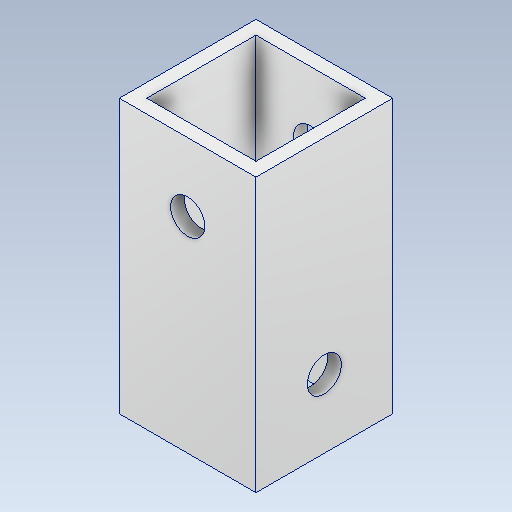
# Autodesk Inventor part: 前後直動12x12x24
Saved by Autodesk Inventor 2020.3 (Build 243373000, 373)
## iProperties
Created: 2020-07-05
Part Number: 前後直動12x12x24
Material: アルミニウム 6061
Document SubType Name: Modeling
Designer: totot
Density: 2.7 g/cm^3
Appearance: アルミニウム - フラット
Author: totot
Autodesk Inventor part; units mm, degrees
ref_plane "YZ Plane" through (0, 0, 0) normal (1, 0, 0) x (0, 1, 0)
ref_plane "XZ Plane" through (0, 0, 0) normal (0, 1, 0) x (-1, 0, 0)
ref_plane "XY Plane" through (0, 0, 0) normal (0, 0, 1) x (1, 0, 0)
sketch "スケッチ1" plane through (0, 0, 0) normal (0, 1, 0) x (-1, 0, 0)
  line L0 (0, 0) -> (12, 0)
  line L1 (12, 0) -> (12, -12)
  line L2 (12, -12) -> (0, -12)
  line L3 (0, -12) -> (0, 0)
  line L4 (1.2, -1.2) -> (10.8, -1.2)
  line L5 (10.8, -1.2) -> (10.8, -10.8)
  line L6 (10.8, -10.8) -> (1.2, -10.8)
  line L7 (1.2, -10.8) -> (1.2, -1.2)
  dimension "d0" = 12
  dimension "d1" = 12
  dimension "d2" = 9.6
  dimension "d3" = 9.6
  dimension "d4" = 1.2
  dimension "d5" = 1.2
  constraints: 16 end point, 4 parallel, 2 horizontal, 2 perpendicular
  measures "d0" distance of L1.end L2.end
  measures "d1" distance of L0.end L1.end
  measures "d2" distance of L5.end L6.end
  measures "d3" distance of L4.end L5.end
  measures "d4" distance between parallel lines of L0 L4
  measures "d5" distance between parallel lines of L7 L3
extrude "押し出し1" add sketch "スケッチ1" along normal blind 24
sketch "スケッチ2" plane through (-12, 0, -12) normal (-1, 0, 0) x (0, 0, 1)
  line L0 (0, 0) -> (12, 0) projected
  line L1 (0, 0) -> (0, 24) projected
  point P0 (6, 6)
  dimension "d8" = 6
  dimension "d9" = 6
  measures "d8" distance from line of point (6, 6) L0
  measures "d9" distance from line of L1 point (6, 6)
hole "穴1" at (-12, 6, -6) direction (1, 0, 0) diameter 3 end through all
sketch "スケッチ3" plane through (0, 0, -12) normal (0, 0, -1) x (-1, 0, 0)
  line L0 (0, 0) -> (0, 24) projected
  line L1 (0, 24) -> (12, 24) projected
  point P0 (6, 18)
  dimension "d17" = 6
  dimension "d18" = 6
  measures "d17" distance from line of L0 point (6, 18)
  measures "d18" distance from line of L1 point (6, 18)
hole "穴2" at (-6, 18, -12) direction (0, 0, 1) diameter 3 end through all
